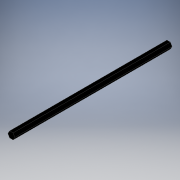
# Autodesk Inventor part: CAR_035_KickerShaft
Saved by Autodesk Inventor 2018 (Build 220112000, 112)
## iProperties
Created: 2020-02-07
Part Number: CAR_035_KickerShaft
Material: Aluminum 6061
Document SubType Name: Modeling
Designer: jd2
Density: 2.7 g/cm^3
Appearance: Aluminum - Flat
Author: jd2
Autodesk Inventor part; units mm, degrees
ref_plane "YZ Plane" through (0, 0, 0) normal (1, 0, 0) x (0, 1, 0)
ref_plane "XZ Plane" through (0, 0, 0) normal (0, 1, 0) x (-1, 0, 0)
ref_plane "XY Plane" through (0, 0, 0) normal (0, 0, 1) x (1, 0, 0)
sketch "Sketch1" plane through (0, 0, 0) normal (0, 0, 1) x (1, 0, 0)
  line L0 (3.6554, 6.3562) -> (7.3323, 0.0125)
  line L1 (7.3323, 0.0125) -> (3.677, -6.3438)
  line L2 (3.677, -6.3438) -> (-3.6554, -6.3562)
  line L3 (-3.6554, -6.3562) -> (-7.3323, -0.0125)
  line L4 (-7.3323, -0.0125) -> (-3.677, 6.3438)
  line L5 (-3.677, 6.3438) -> (3.6554, 6.3562)
  point P0 (0, 0)
  point P1 (0, 0)
  dimension "d0" = 12.7
  constraints: 12 end point, 1 coincident, 13 other
  measures "d0" distance between parallel lines of L2 L5
extrude "Extrusion1" add sketch "Sketch1" along normal blind 330.2
body "Solid1"
